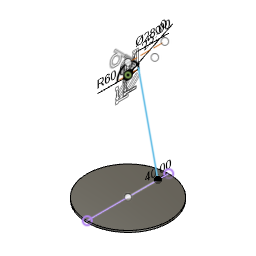
Cannon Base (Autodesk Fusion 360 design; units mm, degrees)
Autodesk Fusion 360 part; units mm, degrees
sketch "Sketch1" plane through (0, 0, 0) normal (0, 0, 1) x (1, 0, 0)
  circle A0 centre (0, 0) radius 150
  dimension "d1" = 300
  constraint coincident A0.centre origin
  measures "d1" diameter of A0
extrude "Extrude1" add sketch "Sketch1" along normal blind 6.2
sketch "Sketch2" plane through (0, 0, 0) normal (1, 0, 0) x (0, 1, 0)
  line L0 (0.0614, 434.8449) -> (0.0614, 436.2)
  line L1 (150, 6.2) -> (-150, 6.2)
  circle A0 centre (0.0614, 395.8449) radius 14
  line L2 (0.0614, 434.8449) -> (135.7194, 434.8449) construction
  line L3 (0.0614, 395.8449) -> (-38.9386, 395.8449) construction
  line L4 (0.0614, 395.8449) -> (39.0614, 395.8449) construction
  line L5 (39.8086, 391.7408) -> (110, 6.2)
  arc A1 (38.9735, 398.4618) -> (-38.9386, 395.8449) centre (0.0614, 395.8449) ccw
  arc A2 (38.9735, 398.4618) -> (39.8086, 391.7408) centre (98.8383, 402.4877) ccw
  line L6 (110, 6.2) -> (0, 6.2)
  dimension "d5" = 28
  dimension "d7" = 25
  dimension "d8" = 40
  dimension "d10" = 60
  constraint vertical L0
  constraint tangent L2 A1
  constraint coincident A0.centre L3.start
  constraint parallel L3 L4
  constraint coincident L1 L5.end
  constraint coincident L4.end L5
  constraint coincident L4.end A1
  constraint tangent A1 A2
  constraint tangent L5 A2
  measures "d5" diameter of A0
  measures "d7" distance of A0 A1
  measures "d8" distance of L1.start L5.end
  measures "d10" radius of A2
